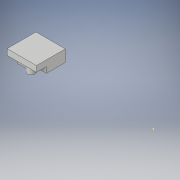
# Autodesk Inventor part: encaixe suporte controlador L
Saved by Autodesk Inventor 2019.4 (Build 234330000, 330)
## iProperties
Created: 2020-12-12
Part Number: encaixe suporte controlador L
Material: Genérico
Document SubType Name: Modeling
Designer: Lattes
Density: 1 g/cm^3
Appearance: Padrão
Author: Lattes
## iProperties of the stored document _3DPrint.ipt
Created: 2020-12-12
Part Number: _3DPrint
Material: Genérico
Document SubType Name: Modeling
Designer: Lattes
Density: 1 g/cm^3
Appearance: Padrão
Author: Lattes
Autodesk Inventor part; units mm, degrees
ref_plane "YZ Plane" through (0, 0, 0) normal (1, 0, 0) x (0, 1, 0)
ref_plane "XZ Plane" through (0, 0, 0) normal (0, 1, 0) x (-1, 0, 0)
ref_plane "XY Plane" through (0, 0, 0) normal (0, 0, 1) x (1, 0, 0)
sketch "Esboço1" plane through (0, 0, 0) normal (0, 1, 0) x (-1, 0, 0)
  line L0 (55, -0.35) -> (55, -10)
  line L1 (67, -0.35) -> (67, -10)
  line L2 (67, -10) -> (55, -10)
  arc A0 (60.65, 1.6525) -> (58.35, 1.6525) centre (59.5, 3) ccw
  line L3 (58.35, 0) -> (58.35, 1.6525)
  line L4 (60.65, 0) -> (60.65, 1.6525)
  line L5 (60.65, 0) -> (60.65, -0.35)
  line L6 (60.65, -0.35) -> (67, -0.35)
  line L7 (58.35, 0) -> (58.35, -0.35)
  line L8 (58.35, -0.35) -> (55, -0.35)
  point P0 (0, 0)
  point P1 (-4, 56.431)
  dimension "d5" = 3.543
  dimension "d8" = 0.35
  constraints: 18 end point, 3 point on line, 2 perpendicular, 2 point on circle, 1 centre point, 1 parallel
  measures "d5" diameter of A0
  measures "d8" distance of L4.start L5.end
extrude "Extrusão1" add sketch "Esboço1" along normal blind 3
sketch "Esboço2" plane through (0, 3, 0) normal (0, 1, 0) x (1, 0, 0)
  point P0 (0, 0)
sketch "Esboço3" plane through (-67, 0, -10) normal (-1, 0, 0) x (0, 0, 1)
  line L0 (9.65, 0) -> (9.65, 3) projected
  line L1 (9.65, 0) -> (9.65, 3)
  line L2 (9.65, 3) -> (0, 3) projected
  line L3 (9.65, 3) -> (0, 3)
  line L4 (0, 0) -> (0, 3) projected
  line L5 (0, 3) -> (0, 0)
  line L6 (0, 0) -> (9.65, 0)
  point P0 (10, 0)
  constraints: 8 end point, 3 perpendicular, 1 vertical
extrude "Extrusão2" add sketch "Esboço3" along normal blind 3
sketch "Esboço4" plane through (0, 3, 0) normal (0, 1, 0) x (1, 0, 0)
  arc A0 (-60.65, -1.6525) -> (-58.35, -1.6525) centre (-59.5, -3) ccw projected
  line L0 (-58.35, 0.35) -> (-55, 0.35) projected
  line L1 (-55, 0.35) -> (-55, -4.7715)
  line L2 (-60.65, 0.35) -> (-70, 0.35) projected
  line L3 (-70, 0.35) -> (-70, -4.7715)
  line L4 (-70, -4.7715) -> (-55, -4.7715)
  line L5 (-70, 0.35) -> (-70, 3.35)
  line L6 (-70, 10) -> (-70, 0.35) projected
  line L7 (-70, 3.35) -> (-55, 3.35)
  line L8 (-55, 3.35) -> (-55, 0.35)
  point P0 (0, 0)
  dimension "d14" = 3
  constraints: 12 end point, 3 perpendicular, 1 point on line, 1 vertical
  measures "d14" distance of L2.end L5.end
extrude "Extrusão3" add sketch "Esboço4" along normal blind 3
sketch "Esboço5" plane through (0, 3, 0) normal (0, 1, 0) x (1, 0, 0)
  line L0 (-70, 10) -> (-55, 10) projected
  line L1 (-70, 3.35) -> (-55, 3.35) projected
  line L2 (-55, 10) -> (-70, 10)
  line L3 (-70, 10) -> (-70, 3.35)
  line L4 (-70, 3.35) -> (-55, 3.35)
  line L5 (-55, 3.35) -> (-55, 10)
  point P0 (0, 0)
  constraints: 8 end point, 2 parallel, 1 horizontal, 1 perpendicular
extrude "Extrusão4" add sketch "Esboço5" along normal blind 3
sketch "Esboço6" plane through (0, 0, 0) normal (0, -1, 0) x (1, 0, 0)
  line L0 (-70, -0.35) -> (-70, 4.7715) projected
  line L1 (-70, -0.35) -> (-65, -0.35)
  line L2 (-60.65, -0.35) -> (-70, -0.35) projected
  line L3 (-65, -0.35) -> (-65, -5.35)
  line L4 (-65, -5.35) -> (-70, -5.35)
  line L5 (-70, -10) -> (-70, -0.35) projected
  line L6 (-70, -0.35) -> (-70, -5.35)
  point P0 (0, 0)
  dimension "d19" = 5
  dimension "d20" = 5
  constraints: 8 end point, 3 perpendicular, 2 point on line
  measures "d19" distance of L0.start L1.end
  measures "d20" distance of L1.end L3.end
extrude "Extrusão5" add sketch "Esboço6" along normal blind 3
chamfer "Chanfro1" distance 3 angle 45 1 edges at (-67.5, 0, -5.35)
